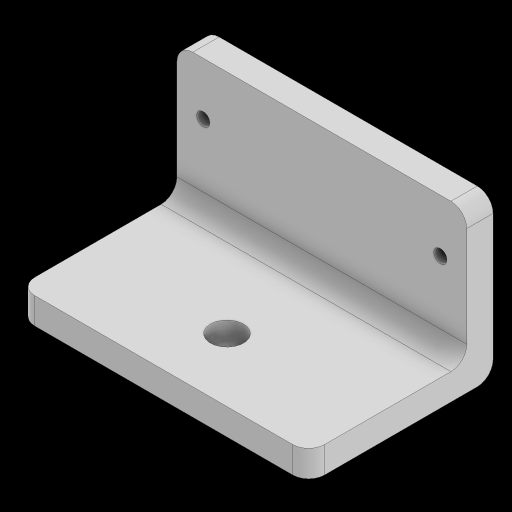
# Autodesk Inventor part: Part1
Saved by Autodesk Inventor 2023 (Build 270158000, 158)
## iProperties
Created: 2025-06-27
Part Number: Part1
Material: 一般
Document SubType Name: Sheet Metal
Designer: Owner
Density: 1 g/cm^3
Sheet Metal Rule: Default_mm
Appearance: 既定
Author: Owner
Autodesk Inventor part; units mm, degrees
ref_plane "YZ Plane" through (0, 0, 0) normal (1, 0, 0) x (0, 1, 0)
ref_plane "XZ Plane" through (0, 0, 0) normal (0, 1, 0) x (-1, 0, 0)
ref_plane "XY Plane" through (0, 0, 0) normal (0, 0, 1) x (1, 0, 0)
sketch "スケッチ1" plane through (0, 0, 0) normal (0, 0, 1) x (1, 0, 0)
  line L0 (-27.5, 25) -> (27.5, 25)
  line L1 (27.5, 25) -> (27.5, 0)
  line L2 (27.5, 0) -> (-27.5, 0)
  line L3 (-27.5, 0) -> (-27.5, 25)
  line L4 (-27.5, 0) -> (27.5, 0)
  line L5 (27.5, 0) -> (27.5, -5)
  line L6 (27.5, -5) -> (-27.5, -5)
  line L7 (-27.5, -5) -> (-27.5, 0)
  circle A0 centre (-22.5, 15) radius 1.25
  line L8 (-27.3778, 15) -> (27.6222, 15)
  line L9 (0, 25) -> (0, -5)
  circle A1 centre (22.5, 15) radius 1.25
  point P0 (0, 0)
  point P1 (0, 0)
  point P2 (0, 0)
  dimension "d0" = 25
  dimension "d1" = 55
  dimension "d2" = 5
  dimension "d4" = 22.5
  dimension "d5" = 2.5
  dimension "d17" = 10
  constraints: 20 end point, 4 midpoint, 4 parallel, 3 perpendicular, 2 centre point, 2 horizontal, 1 coincident, 1 point on line, 1 symmetric about line, 1 other
  measures "d0" distance of L0.end L1.end
  measures "d1" distance of L1.end L2.end
  measures "d2" distance of L6.end L2.end
  measures "d4" horizontal distance of point (0, 0) A0.centre
  measures "d5" diameter of A0
  measures "d17" vertical distance of L0.start L8.start
extrude "押し出し1" add sketch "スケッチ1" along normal blind 5 contours L0 L9 L2 L3 | L0 L1 L8 A1 L9 | L8 A1 L1 L2 L9
extrude "押し出し2" add sketch "スケッチ1" along normal blind 35 contours L2 L9 L6 L7 | L2 L5 L6 L9
sketch "スケッチ2" plane through (-27.5, -5, 0) normal (0, -1, 0) x (1, 0, 0)
  line L0 (0, 35) -> (55, 35) projected
  line L1 (54.9263, 23) -> (-0.0737, 23)
  line L2 (27.5, 35) -> (27.5, 0)
  circle A0 centre (27.5, 23) radius 3.15
  dimension "d15" = 6.3
  dimension "d18" = 12
  constraints: 4 end point, 2 point on line, 1 centre point, 1 midpoint, 1 perpendicular
  measures "d15" diameter of A0
  measures "d18" distance between parallel lines of L0 L1
extrude "押し出し3" cut sketch "スケッチ2" against normal blind 30
fillet "フィレット1" radius 3 2 edges at (0, -5, 0) (0, 0, 5)
fillet "フィレット2" radius 3 4 edges at (27.5, -2.5, 35) (-27.5, -2.5, 35) (27.5, 25, 2.5) (-27.5, 25, 2.5)
equation "\"BendRadius\" = Thickness"
equation "\"BendReliefWidth\" = Thickness"
equation "\"BendReliefDepth\" = 0.5 * Thickness"
equation "\"CornerReliefSize\" = 4 * Thickness"
equation "\"MinimumRemnant\" = 2 * Thickness"
equation "\"TransitionRadius\" = BendRadius"
equation "\"JacobiRadiusSize\" = BendRadius"
equation "\"GapSize\" = Thickness"
equation "\"Thickness\" = 0.5"
